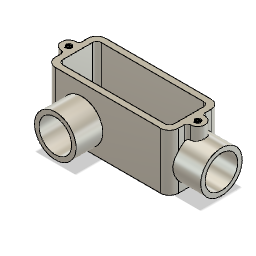
Part2Conduit v2 (Autodesk Fusion 360 design; units mm, degrees)
Autodesk Fusion 360 part; units mm, degrees
sketch "Sketch1" plane through (0, 0, 0) normal (0, 1, 0) x (1, 0, 0) in component "Body"
  line L0 (41.5, 17) -> (-41.5, 17)
  line L1 (-41.5, 17) -> (-41.5, -17)
  line L2 (-41.5, -17) -> (41.5, -17)
  line L3 (41.5, -17) -> (41.5, 17)
  line L4 (41.5, 17) -> (-41.5, -17) construction
  line L5 (-41.5, 17) -> (41.5, -17) construction
  dimension "d1" = 83
  dimension "d2" = 34
  constraint horizontal L0
  constraint perpendicular L0 L1
  constraint parallel L0 L2
  constraint parallel L1 L3
  constraint coincident L4 origin
  constraint coincident L5 origin
  measures "d1" distance of L1.end L2.end
  measures "d2" distance of L0.end L1.end
extrude "Extrude1" add sketch "Sketch1" along normal blind 38
sketch "Sketch1 (2)" plane through (0, 38, 0) normal (0, 1, 0) x (-1, 0, 0)
  line L0 (-41.5, 17) -> (-41.5, -17)
  line L1 (-41.5, -17) -> (41.5, -17)
  line L2 (41.5, -17) -> (41.5, 17)
  line L3 (41.5, 17) -> (-41.5, 17)
  line L4 (37.5, 13) -> (-37.5, 13)
  line L5 (-37.5, 13) -> (-37.5, -13)
  line L6 (-37.5, -13) -> (37.5, -13)
  line L7 (37.5, -13) -> (37.5, 13)
  dimension "d5" = -4
extrude "Extrude2" cut sketch "Sketch1 (2)" against normal up to surface (34 mm away) contours L4 L5 L6 L7
fillet "Fillet1" radius 3 4 edges at (-37.5, 21, -13) (-37.5, 21, 13) (37.5, 21, -13) (37.5, 21, 13)
fillet "Fillet2" radius 6 4 edges at (-41.5, 19, 17) (41.5, 19, -17) (41.5, 19, 17) (-41.5, 19, -17)
sketch "Sketch2" plane through (0, 0, 17) normal (0, 0, 1) x (1, 0, 0)
  line L0 (35.5, 0) -> (35.5, 38)
  line L1 (35.5, 38) -> (-35.5, 38)
  line L2 (-35.5, 38) -> (-35.5, 0)
  line L3 (-35.5, 0) -> (35.5, 0)
  circle A0 centre (-17.5, 16) radius 14
  line L4 (-41.5, 38) -> (-41.5, 0)
  dimension "d12" = 28
  dimension "d13" = 24
  dimension "d14" = 16
  measures "d12" diameter of A0
  measures "d13" distance of A0.centre L4
  measures "d14" distance of L3 A0.centre
extrude "Extrude3" add sketch "Sketch2" along normal blind 18 contours A0
sketch "Sketch3" plane through (0, 0, 35) normal (0, 0, 1) x (1, 0, 0)
  circle A0 centre (-17.5, 16) radius 14
  circle A1 centre (-17.5, 16) radius 11
  dimension "d17" = 22
  constraint concentric A0 A1
  measures "d17" diameter of A1
extrude "Extrude4" cut sketch "Sketch3" against normal up to surface (22 mm away) contours A1
sketch "Sketch4" plane through (41.5, 0, 0) normal (1, 0, 0) x (0, 0, -1)
  line L0 (-11, 38) -> (-11, 0)
  line L1 (-11, 0) -> (11, 0)
  line L2 (11, 0) -> (11, 38)
  line L3 (11, 38) -> (-11, 38)
  line L4 (0, 0) -> (0, 44.7494) construction
  circle A0 centre (0, 16) radius 14
  dimension "d20" = 28
  dimension "d21" = 16
  constraint coincident L4.start origin
  constraint perpendicular L3 L4
  constraint coincident L4 A0.centre
  measures "d20" diameter of A0
  measures "d21" distance of L1 A0.centre
extrude "Extrude5" add sketch "Sketch4" along normal up to surface (-4 mm away) and the other way blind -18 contours L0 L2 A0 | L0 A0 | L2 A0
sketch "Sketch5" plane through (59.5, 0, 0) normal (1, 0, 0) x (0, 0, -1)
  circle A0 centre (0, 16) radius 14
  circle A1 centre (0, 16) radius 11
  dimension "d32" = -3
sketch "Sketch6" plane through (0, 38, 0) normal (0, 1, 0) x (-1, 0, 0)
  arc A0 (35.5, -17) -> (41.5, -11) centre (35.5, -11) ccw
  line L0 (41.5, -11) -> (41.5, 11)
  arc A1 (41.5, 11) -> (35.5, 17) centre (35.5, 11) ccw
  line L1 (35.5, 17) -> (-35.5, 17)
  arc A2 (-35.5, 17) -> (-41.5, 11) centre (-35.5, 11) ccw
  line L2 (-41.5, 11) -> (-41.5, -11)
  arc A3 (-41.5, -11) -> (-35.5, -17) centre (-35.5, -11) ccw
  line L3 (-35.5, -17) -> (35.5, -17)
  line L4 (34.5, -13) -> (-34.5, -13)
  arc A4 (-37.5, -10) -> (-34.5, -13) centre (-34.5, -10) ccw
  line L5 (-37.5, -10) -> (-37.5, 10)
  arc A5 (-34.5, 13) -> (-37.5, 10) centre (-34.5, 10) ccw
  line L6 (-34.5, 13) -> (34.5, 13)
  arc A6 (37.5, 10) -> (34.5, 13) centre (34.5, 10) ccw
  line L7 (37.5, 10) -> (37.5, -10)
  arc A7 (34.5, -13) -> (37.5, -10) centre (34.5, -10) ccw
  line L8 (0, 0) -> (52.9158, 0) construction
  circle A8 centre (43.5, 0) radius 5
  dimension "d35" = 10
  dimension "d36" = 6
  constraint coincident L8.start origin
  constraint perpendicular L7 L8
  constraint coincident L8 A8.centre
  measures "d35" diameter of A8
  measures "d36" distance of L7 A8.centre
extrude "Extrude7" add sketch "Sketch6" against normal blind 21 contours L0 A8 picked at (44.0389, 0.1564)
mirror "Mirror1" about plane through (0, 0, 0) normal (1, 0, 0) of "Extrude7"
extrude "Extrude6" cut sketch "Sketch5" against normal up to surface (22 mm away) contours A1
fillet "Fillet3" radius 2 4 edges at (41.5, 33.6144, 4.5826) (41.5, 33.6144, -4.5826) (-41.5, 27.5, -4.5826) (-41.5, 27.5, 4.5826)
sketch "Sketch7" plane through (0, 38, 0) normal (0, 1, 0) x (-1, 0, 0)
  arc A0 (35.5, -17) -> (41.5, -11) centre (35.5, -11) ccw
  line L0 (41.5, -11) -> (41.5, -7)
  arc A1 (43.5, -5) -> (41.5, -7) centre (43.5, -7) ccw
  arc A2 (43.5, -5) -> (43.5, 5) centre (43.5, 0) ccw
  arc A3 (41.5, 7) -> (43.5, 5) centre (43.5, 7) ccw
  line L1 (41.5, 7) -> (41.5, 11)
  arc A4 (41.5, 11) -> (35.5, 17) centre (35.5, 11) ccw
  line L2 (35.5, 17) -> (-35.5, 17)
  arc A5 (-35.5, 17) -> (-41.5, 11) centre (-35.5, 11) ccw
  line L3 (-41.5, 11) -> (-41.5, 7)
  arc A6 (-43.5, 5) -> (-41.5, 7) centre (-43.5, 7) ccw
  arc A7 (-43.5, 5) -> (-43.5, -5) centre (-43.5, 0) ccw
  arc A8 (-41.5, -7) -> (-43.5, -5) centre (-43.5, -7) ccw
  line L4 (-41.5, -7) -> (-41.5, -11)
  arc A9 (-41.5, -11) -> (-35.5, -17) centre (-35.5, -11) ccw
  line L5 (-35.5, -17) -> (35.5, -17)
  line L6 (34.5, -13) -> (-34.5, -13)
  arc A10 (-37.5, -10) -> (-34.5, -13) centre (-34.5, -10) ccw
  line L7 (-37.5, -10) -> (-37.5, 10)
  arc A11 (-34.5, 13) -> (-37.5, 10) centre (-34.5, 10) ccw
  line L8 (-34.5, 13) -> (34.5, 13)
  arc A12 (37.5, 10) -> (34.5, 13) centre (34.5, 10) ccw
  line L9 (37.5, 10) -> (37.5, -10)
  arc A13 (34.5, -13) -> (37.5, -10) centre (34.5, -10) ccw
  circle A14 centre (43.5, 0) radius 2
  circle A15 centre (-43.5, 0) radius 2
  dimension "d43" = 4
  dimension "d47" = 4
  constraint concentric A2 A14
  constraint concentric A7 A15
  measures "d43" diameter of A14
  measures "d47" diameter of A15
extrude "Extrude8" cut sketch "Sketch7" against normal blind 8 contours A14 | A15
thread "Thread1" "ISO Metric profile 4.0 M4x0.7 6H" major diameter 4.1095 minor diameter 3.332 pitch 0.7 angle 60 modelled right hand crest width 0.193 on face at (-45.4901, 35.3333, -0.1991) crest through (-45.166, 37.825, 0) on face at (41.5099, 35.3333, -0.1991) crest through (41.834, 37.825, 0)
component "Body" placed x (1, 0, 0) y (0, 1, 0) z (0, 0, 1) at (0, 0, 0)
component "Lid" placed x (1, 0, 0) y (0, 1, 0) z (0, 0, 1) at (0, 0, 0)
